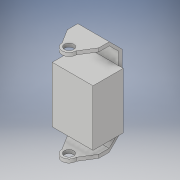
# Autodesk Inventor part: Cversion2
Saved by Autodesk Inventor 2018 (Build 220112000, 112)
## iProperties
Created: 2021-03-23
Part Number: Cversion2
Material: Generic
Document SubType Name: Modeling
Designer: Familia
Density: 1 g/cm^3
Appearance: Default
Author: Familia
Autodesk Inventor part; units mm, degrees
ref_plane "YZ Plane" through (0, 0, 0) normal (1, 0, 0) x (0, 1, 0)
ref_plane "XZ Plane" through (0, 0, 0) normal (0, 1, 0) x (-1, 0, 0)
ref_plane "XY Plane" through (0, 0, 0) normal (0, 0, 1) x (1, 0, 0)
sketch "Sketch1" plane through (0, 0, 0) normal (0, 0, 1) x (1, 0, 0)
  circle A0 centre (0, 0) radius 4
  arc A1 (-6, 0) -> (6, 0) centre (0, 0) ccw
  line L0 (0, 21) -> (13.5, 21)
  line L1 (13.5, 21) -> (-13.5, 21)
  line L2 (-13.5, 21) -> (-13.5, 12)
  line L3 (-13.5, 12) -> (-6, 0)
  line L4 (13.5, 21) -> (13.5, 12)
  line L5 (13.5, 12) -> (6, 0)
  dimension "d0" = 8
  dimension "d1" = 12
  dimension "d2" = 21
  dimension "d3" = 13.5
  dimension "d4" = 27
  dimension "d5" = 9
  dimension "d6" = 9
  constraints: 12 end point, 2 centre point, 2 coincident, 2 point on circle, 1 parallel, 1 perpendicular, 1 point on line
  measures "d0" diameter of A0
  measures "d1" diameter of A1
  measures "d2" distance of A1.centre L0.start
  measures "d3" distance of L0.start L0.end
  measures "d4" distance of L0.end L1.end
  measures "d5" distance of L1.end L2.end
  measures "d6" distance of L0.end L4.end
extrude "Extrusion1" add sketch "Sketch1" along normal blind 3
sketch "Sketch2" plane through (13.5, 12, 0) normal (1, 0, 0) x (0, 0, -1)
  line L0 (8, 20) -> (-3, 9)
  line L1 (8, 20) -> (68, 20)
  line L2 (79, 9) -> (68, 20)
  line L3 (0, 9) -> (-3, 9) projected
  line L4 (-3, 9) -> (0, 9)
  line L5 (0, 9) -> (8, 17)
  line L6 (79.1439, 8.8561) -> (76.1439, 8.8561)
  line L7 (76.1439, 8.8561) -> (68, 17)
  line L8 (39.224, 17) -> (8, 17)
  line L9 (39.224, 17) -> (68, 17)
  line L10 (-3, 0) -> (-3, -12) projected
  line L11 (8, 17) -> (68, 17)
  line L12 (-3, 9) -> (0, 9)
  line L13 (0, 9) -> (8, 17)
  line L14 (8, 17) -> (68, 17)
  line L15 (76.1439, 8.8561) -> (79.1439, 8.8561)
  line L16 (79.1439, 8.8561) -> (68, 20)
  line L17 (68, 20) -> (8, 20)
  line L18 (8, 20) -> (-3, 9)
  line L19 (-3, 9) -> (0, 9)
  point P0 (0, -12)
  dimension "d11" = 60
  dimension "d14" = 3
  constraints: 36 end point, 6 collinear, 4 horizontal, 3 parallel
  measures "d11" distance of L0.start L1.end
  measures "d14" distance of L6.start L6.end
extrude "Extrusion2" add sketch "Sketch2" against normal blind 27
sketch "Sketch3" plane through (13.5, 20.8561, -79.1439) normal (0, -1, 0) x (1, 0, 0)
  line L0 (0, 0) -> (-27, 0) projected
  line L1 (0, 0) -> (-27, 0)
  line L2 (0, 3) -> (-27, 3) projected
  line L3 (-27, 0) -> (-27, 3)
  line L4 (-27, 3) -> (0, 3)
  line L5 (0, 3) -> (0, 0)
  point P0 (-13.5, 79.1439)
  constraints: 8 end point, 3 perpendicular, 1 horizontal
extrude "Extrusion3" add sketch "Sketch3" along normal blind 45
sketch "Sketch4" plane through (13.5, 29, -68) normal (0, -1, 0) x (1, 0, 0)
  line L0 (0, 0) -> (0, 60) projected
  line L1 (0, 1.254) -> (-27, 1.254)
  line L2 (-27, 0) -> (-27, 60) projected
  line L3 (0, 1.254) -> (-13.5, 1.254)
  line L4 (-13.5, 1.254) -> (4, 1.254)
  line L5 (4, 1.254) -> (4, 49.254)
  line L6 (4, 49.254) -> (-31, 49.254)
  line L7 (-31, 49.254) -> (-31, 1.254)
  line L8 (-31, 1.254) -> (4, 1.254)
  point P0 (-13.5, 68)
  dimension "d20" = 1.254
  dimension "d21" = 17.5
  dimension "d22" = 48
  dimension "d23" = 35
  constraints: 14 end point, 4 point on line, 3 perpendicular, 1 collinear, 1 midpoint
  measures "d20" distance of L0.start L1.start
  measures "d21" distance of L3.end L4.end
  measures "d22" distance of L4.end L5.end
  measures "d23" distance of L5.end L6.end
extrude "Extrusion4" add sketch "Sketch4" along normal blind 26
sketch "Sketch5" plane through (13.5, 32, -8) normal (0, 1, 0) x (1, 0, 0)
  line L0 (-27, 0) -> (-27, 60) projected
  line L1 (0, 60) -> (-27, 60) projected
  circle A0 centre (-13.5, 46.746) radius 4
  point P0 (-13.5, -8)
  dimension "d28" = 8
  constraints: 1 centre point
  measures "d28" diameter of A0
extrude "Extrusion5" add sketch "Sketch5" along normal blind 10
sketch "Sketch6" plane through (13.5, 20.8561, -79.1439) normal (0, 0, -1) x (-1, 0, 0)
  circle A0 centre (13.5, -21) radius 4
  arc A1 (7.5004, -20.9281) -> (19.4996, -20.9281) centre (13.5, -21) ccw
  line L0 (27, -9) -> (19.5, -21)
  line L1 (7.5, -20.8561) -> (0, -8.8561) projected
  line L2 (0, -8.8561) -> (7.5, -20.8561)
  line L3 (27, 0) -> (27, -45) projected
  line L4 (27, -9) -> (27, -45)
  line L5 (0, -45) -> (27, -45) projected
  line L6 (27, -45) -> (0, -45)
  line L7 (0, -45) -> (0, -8.8561)
  arc A2 (7.5, -20.8561) -> (19.5, -20.8561) centre (13.5, -20.8561) ccw projected
  arc A3 (7.5, -20.8561) -> (19.5, -20.8561) centre (13.5, -21) ccw
  point P0 (0, 0.1439)
  dimension "d34" = 8
  dimension "d35" = 12
  constraints: 10 end point, 9 point on circle, 3 centre point, 3 collinear, 2 coincident, 1 perpendicular
  measures "d34" diameter of A0
  measures "d35" diameter of A1
extrude "Extrusion6" cut sketch "Sketch6" against normal blind 4 contours A0 | A1 L0 L3 L5 L7 L1 A2
body "Solid1"
